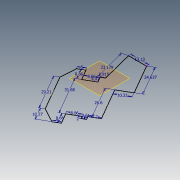
# Autodesk Inventor part: Upper Support
Saved by Autodesk Inventor 2014 SP1 (Build 180222100, 222)
## iProperties
Created: 2014-04-03
Part Number: Upper Support
Material: Generic
Document SubType Name: Modeling
Designer: tom
Density: 1 g/cm^3
Appearance: Default
Author: tom
Autodesk Inventor part; units mm, degrees
ref_plane "YZ Plane" through (0, 0, 0) normal (1, 0, 0) x (0, 1, 0)
ref_plane "XZ Plane" through (0, 0, 0) normal (0, 1, 0) x (-1, 0, 0)
ref_plane "XY Plane" through (0, 0, 0) normal (0, 0, 1) x (1, 0, 0)
ref_plane "Work Plane3" through (-98.2192, 25.6748, -72.651) normal (0, 1, 0) x (1, 0, 0)
sketch "Sketch1" plane through (-98.2192, 25.6748, -72.651) normal (0, 1, 0) x (1, 0, 0)
  line L0 (108.2722, -112.7231) -> (109.1382, -112.2231) construction
  line L1 (108.6382, -111.3571) -> (109.1382, -112.2231) construction
  line L2 (101.5917, -99.1522) -> (114.8917, -122.1885)
  line L3 (101.5917, -99.1522) -> (110.5377, -93.9872)
  line L4 (114.8917, -122.1885) -> (108.6563, -125.7885)
  line L5 (108.6563, -125.7885) -> (109.9613, -128.0488)
  line L6 (109.9613, -128.0488) -> (107.3632, -129.5488)
  line L7 (107.3632, -129.5488) -> (106.3632, -127.8168)
  line L8 (106.3632, -127.8168) -> (98.8635, -132.1468)
  line L9 (98.8635, -132.1468) -> (103.1935, -139.6466)
  line L10 (79.4712, -121.2385) -> (82.4842, -126.4571) construction
  line L11 (103.1935, -139.6466) -> (98.8633, -142.1466)
  line L12 (83.0235, -104.7111) -> (90.5232, -100.3811)
  line L13 (90.5232, -100.3811) -> (88.3182, -96.5619)
  line L14 (88.3182, -96.5619) -> (90.8427, -95.1044)
  line L15 (83.0235, -104.7111) -> (78.6935, -97.2113)
  line L16 (73.6327, -111.1259) -> (88.2377, -136.4225)
  line L17 (78.6935, -97.2113) -> (74.3633, -99.7113)
  line L18 (90.8427, -95.1044) -> (85.0892, -72.651)
  line L19 (110.5377, -93.9872) -> (98.2192, -72.651)
  line L20 (98.2192, -72.651) -> (85.0892, -72.651)
  line L21 (88.2377, -136.4225) -> (98.8633, -142.1466)
  line L22 (74.3633, -99.7113) -> (73.6327, -111.1259)
  dimension "d1" = 26.6
  dimension "d4" = 7.2
  dimension "d5" = 2.61
  dimension "d6" = 3
  dimension "d7" = 2
  dimension "d8" = 8.66
  dimension "d9" = 8.66
  dimension "d10" = 5
  dimension "d11" = 8.66
  dimension "d12" = 31.68
  dimension "d13" = 4.41
  dimension "d14" = 2.915
  dimension "d17" = 8.66
  dimension "d18" = 29.21
  dimension "d20" = 10.27
  dimension "d21" = 5
  dimension "d22" = 23.1789
  dimension "d23" = 13.13
  dimension "d24" = 24.637
  dimension "d25" = 10.33
  constraints: 46 end point, 7 perpendicular, 1 collinear, 1 parallel
  measures "d1" distance of L2.start L2.end
  measures "d4" distance of L2.end L4.end
  measures "d5" distance of L4.end L5.end
  measures "d6" distance of L5.end L6.end
  measures "d7" distance of L6.end L7.end
  measures "d8" distance of L7.end L8.end
  measures "d9" distance of L8.end L9.end
  measures "d10" distance of L9.end L11.end
  measures "d11" distance of L12.start L12.end
  measures "d12" distance between parallel lines of L8 L12
  measures "d13" distance of L12.end L13.end
  measures "d14" distance of L13.end L14.end
  measures "d17" distance of L12.start L15.end
  measures "d18" distance of L16.start L16.end
  measures "d20" distance from line of L11 L16.end
  measures "d21" distance of L15.end L17.end
  measures "d22" distance of L14.end L18.end
  measures "d23" distance of L19.end L18.end
  measures "d24" distance of L3.end L19.end
  measures "d25" distance of L2.start L3.end
extrude "Extrusion1" add sketch "Sketch1" along normal blind 8.66
body "Solid1"
